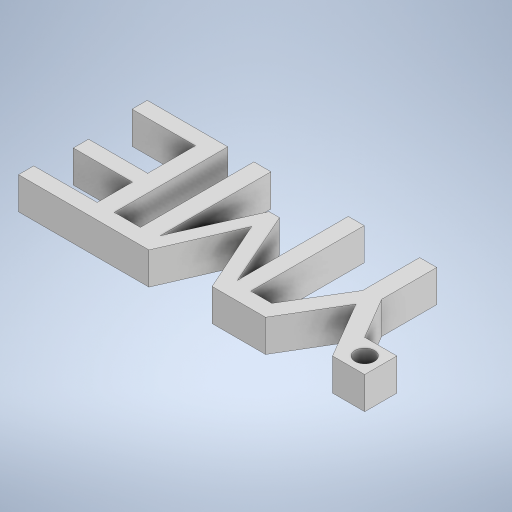
# Autodesk Inventor part: YME
Saved by Autodesk Inventor 2023 (Build 270158000, 158)
## iProperties
Created: 2023-11-27
Part Number: YME
Material: Generic
Document SubType Name: Modeling
Designer: Mustapha
Density: 1 g/cm^3
Appearance: Default
Author: Mustapha
Autodesk Inventor part; units mm, degrees
ref_plane "YZ Plane" through (0, 0, 0) normal (1, 0, 0) x (0, 1, 0)
ref_plane "XZ Plane" through (0, 0, 0) normal (0, 1, 0) x (-1, 0, 0)
ref_plane "XY Plane" through (0, 0, 0) normal (0, 0, 1) x (1, 0, 0)
sketch "Sketch1" plane through (0, 0, 0) normal (0, 1, 0) x (-1, 0, 0)
  line L0 (4.0726, -0.3796) -> (56.5523, -0.3796) construction
  line L1 (56.5523, -0.3796) -> (56.5523, -20.3796) construction
  line L2 (56.5523, -20.3796) -> (4.0726, -20.3796) construction
  line L3 (4.0726, -20.3796) -> (4.0726, -0.3796) construction
  line L4 (20.1018, -0.3796) -> (13.3433, -11.5303)
  line L5 (13.3433, -11.5303) -> (13.3433, -20.3796)
  line L6 (13.3433, -20.3796) -> (10.6852, -20.3796)
  line L7 (10.6852, -20.3796) -> (10.6852, -11.8059)
  line L8 (10.6852, -11.8059) -> (3.9267, -0.3796)
  line L9 (3.9267, -0.3796) -> (6.8765, -0.3796)
  line L10 (6.8765, -0.3796) -> (12.0305, -9.1803)
  line L11 (12.0305, -9.1803) -> (17.2817, -0.3796)
  line L12 (17.2817, -0.3796) -> (20.1018, -0.3796)
  line L13 (39.0969, -20.3796) -> (36.4389, -20.3796)
  line L14 (36.4389, -20.3796) -> (36.4389, -3.1511)
  line L15 (36.4389, -3.1511) -> (31.2201, -14.8691)
  line L16 (31.2201, -14.8691) -> (29.5993, -14.8691)
  line L17 (29.5993, -14.8691) -> (24.4292, -3.1511)
  line L18 (24.4292, -3.1511) -> (24.4292, -20.3796)
  line L19 (24.4292, -20.3796) -> (21.9494, -20.3796)
  line L20 (21.9494, -20.3796) -> (21.9494, -0.3796)
  line L21 (21.9494, -0.3796) -> (25.5799, -0.3796)
  line L22 (25.5799, -0.3796) -> (30.5718, -11.5141)
  line L23 (30.5718, -11.5141) -> (35.4016, -0.3796)
  line L24 (35.4016, -0.3796) -> (39.0969, -0.3796)
  line L25 (39.0969, -0.3796) -> (39.0969, -20.3796)
  line L26 (43.1488, -20.3796) -> (43.1488, -0.3796)
  line L27 (43.1488, -0.3796) -> (55.6609, -0.3796)
  line L28 (55.6609, -0.3796) -> (55.6609, -2.7459)
  line L29 (55.6609, -2.7459) -> (45.8068, -2.7459)
  line L30 (45.8068, -2.7459) -> (45.8068, -8.224)
  line L31 (45.8068, -8.224) -> (54.9964, -8.224)
  line L32 (54.9964, -8.224) -> (54.9964, -10.5903)
  line L33 (54.9964, -10.5903) -> (45.8068, -10.5903)
  line L34 (45.8068, -10.5903) -> (45.8068, -18.0133)
  line L35 (45.8068, -18.0133) -> (55.6609, -18.0133)
  line L36 (55.6609, -18.0133) -> (55.6609, -20.3796)
  line L37 (55.6609, -20.3796) -> (43.1488, -20.3796)
  point P0 (0, 0)
  constraints: 2 other
extrude "Extrusion1" add sketch "Sketch1" along normal blind 5
sketch "Sketch2" plane through (0, 5, 0) normal (0, 1, 0) x (1, 0, 0)
  line L0 (-17.2817, 0.3796) -> (-12.0305, 9.1803) projected
  line L1 (-55.6609, 0.3796) -> (-43.1488, 0.3796) projected
  line L2 (-17.2817, 0.3796) -> (-20.1018, 0.3796)
  line L3 (-55.6609, 2.7459) -> (-55.6609, 0.3796) projected
  line L4 (-55.6609, 0.3796) -> (-55.6609, 2.7459)
  line L5 (-55.6609, 2.7459) -> (-16.2934, 2.7459)
  line L6 (-16.2934, 2.7459) -> (-17.3426, 0.3796)
  line L7 (-13.3433, 11.5303) -> (-20.1018, 0.3796) projected
  line L8 (-20.1018, 0.3796) -> (-24.9933, 0.3796)
  line L9 (-21.9494, 0.3796) -> (-25.5799, 0.3796) projected
  line L10 (-26.1142, 2.7459) -> (-24.9933, 0.3796)
  line L11 (-55.6609, 0.3796) -> (-38.2567, 0.3796)
  line L12 (-39.0969, 0.3796) -> (-35.4016, 0.3796) projected
  line L13 (-38.2567, 2.7459) -> (-49.9322, 2.7459)
  line L14 (-38.2567, 0.3796) -> (-38.2567, 2.7459)
  point P0 (0, 0)
  constraints: 18 end point, 7 point on line, 3 perpendicular, 1 collinear
extrude "Extrusion2" add sketch "Sketch2" against normal blind 5
sketch "Sketch3" plane through (0, 5, 0) normal (0, 1, 0) x (1, 0, 0)
  line L0 (-6.8765, 0.3796) -> (-3.9267, 0.3796) projected
  line L1 (-6.8765, 0.3796) -> (-1.8765, 0.3796)
  line L2 (-1.8765, 0.3796) -> (-1.8765, 5.3796)
  line L3 (-1.8765, 5.3796) -> (-6.8765, 5.3796)
  line L4 (-6.8765, 5.3796) -> (-6.8765, 0.3796)
  point P0 (0, 0)
  dimension "d9" = 5
  dimension "d10" = 5
  constraints: 8 end point, 2 parallel, 1 horizontal, 1 perpendicular
  measures "d9" distance between parallel lines of L1 L3
  measures "d10" distance between parallel lines of L2 L4
extrude "Extrusion3" add sketch "Sketch3" against normal blind 5
sketch "Sketch4" plane through (0, 5, 0) normal (0, 1, 0) x (1, 0, 0)
  circle A0 centre (-4.3765, 2.8796) radius 1.5
  line L0 (-6.8765, 0.3796) -> (-1.8765, 0.3796) projected
  line L1 (-1.8765, 0.3796) -> (-1.8765, 5.3796) projected
  point P0 (0, 0)
  dimension "d6" = 2.5
  dimension "d11" = 2.5
  dimension "d12" = 3
  constraints: 1 centre point
  measures "d6" distance from line of A0.centre L0
  measures "d11" distance from line of L1 A0.centre
  measures "d12" diameter of A0
extrude "Extrusion4" cut sketch "Sketch4" against normal blind 5
body "Solid1"
